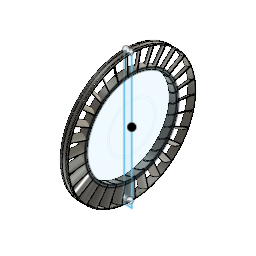
petrol_turbine_two_eng_model (Autodesk Fusion 360 design; units mm, degrees)
Autodesk Fusion 360 part; units mm, degrees
sketch "Sketch1" plane through (0, 0, 0) normal (1, 0, 0) x (0, 1, 0)
  circle A0 centre (0, 0) radius 58.75
  circle A1 centre (0, 0) radius 63.75
  dimension "d1" = 117.5
  dimension "d2" = 5
  constraint coincident A0.centre A1.centre
  measures "d1" diameter of A0
  measures "d2" distance of A0 A1
extrude "Extrude1" add sketch "Sketch1" along normal blind 20 makes body 1
sketch "Sketch2" plane through (0, 0, 0) normal (0, 1, 0) x (1, 0, 0)
  line L0 (0, -63.75) -> (0, 63.75)
  line L1 (20, -63.75) -> (20, 63.75)
  line L2 (0, 0) -> (0, -268.9117) construction
  line L3 (20, 0) -> (20, -259.4819) construction
  line L4 (0, -166.64) -> (20, -166.64)
  line L5 (0, -166.64) -> (0, -168.64)
  line L6 (20, -166.64) -> (20, -168.64)
  arc A0 (4, -168.64) -> (6, -168.64) centre (5, -168.64) ccw
  line L7 (0, -168.64) -> (4, -168.64)
  arc A1 (14, -168.64) -> (16, -168.64) centre (15, -168.64) ccw
  line L8 (6, -168.64) -> (14, -168.64)
  line L9 (16, -168.64) -> (20, -168.64)
  dimension "d5" = 166.64
  dimension "d6" = 166.64
  dimension "d8" = 2
  dimension "d9" = 2
  dimension "d10" = 5
  dimension "d11" = 5
  constraint coincident L2.start origin
  constraint parallel L0 L2
  constraint midpoint L1 L3.start
  constraint parallel L1 L3
  constraint coincident L2 L4.start
  constraint coincident L3 L4.end
  constraint coincident A0.centre L7
  constraint coincident A1.centre L7
  constraint coincident A0.end L7
  constraint collinear L7 L8
  constraint coincident A1.end L8
  constraint collinear L8 L9
  measures "d5" distance of L3.start L4.end
  measures "d6" distance of L2.start L4.start
  measures "d8" diameter of A0
  measures "d9" diameter of A1
  measures "d10" distance of L5.end A0.centre
  measures "d11" distance of L3 A1.centre
revolve "Revolve1" add sketch "Sketch2" angle 360 about axis through (1.75, 0, 0) along (1, 0, 0) separate body makes body 2
sketch "Sketch3" plane through (0, 0, 0) normal (0, 1, 0) x (1, 0, 0)
  line L0 (20, 168.64) -> (20, -168.64)
  line L1 (0, 168.64) -> (0, -168.64)
  line L2 (20, 168.64) -> (16, 168.64)
  line L3 (20, -168.64) -> (16, -168.64)
  arc A0 (14, -168.64) -> (16, -168.64) centre (15, -168.64) ccw
  arc A1 (16, 168.64) -> (14, 168.64) centre (15, 168.64) ccw
  line L4 (14, 168.64) -> (6, 168.64)
  line L5 (14, -168.64) -> (6, -168.64)
  arc A2 (4, -168.64) -> (6, -168.64) centre (5, -168.64) ccw
  arc A3 (6, 168.64) -> (4, 168.64) centre (5, 168.64) ccw
  line L6 (4, 168.64) -> (0, 168.64)
  line L7 (4, -168.64) -> (0, -168.64)
  line L8 (0, 168.64) -> (0, 183.603)
  line L9 (20, 168.64) -> (20, 183.603)
  line L10 (0, 183.603) -> (20, 183.603)
  constraint perpendicular L6 L8
  constraint perpendicular L2 L9
  constraint perpendicular L9 L10
sketch "Sketch4" plane through (0, 0, 0) normal (0, 0, 1) x (1, 0, 0)
  line L0 (0, 0) -> (74.0106, 0) construction
  line L1 (20, 168.64) -> (20, -168.64) construction
  line L2 (20, 0) -> (16, 0) construction
  arc A0 (19.8633, -9.4953) -> (2.0217, 0.9998) centre (1.5616, -20.1952) ccw
  arc A1 (18.1367, -10.5047) -> (1.9783, -0.9998) centre (1.5616, -20.1952) ccw
  line L3 (1.9783, -0.9998) -> (2.0217, 0.9998)
  line L4 (18.1367, -10.5047) -> (19.8633, -9.4953)
  point P0 (2, 0)
  point P1 (19, -10)
  dimension "d13" = 2
  dimension "d14" = 1
  dimension "d15" = 10
  constraint coincident L0.start origin
  constraint horizontal L0
  constraint coincident L0 P0
  measures "d13" distance of L0.start P0
  measures "d14" distance of P1 L1
  measures "d15" distance of P1 L2
extrude "Extrude2" add sketch "Sketch4" along normal blind 168 separate body makes body 3
fillet "Fillet1" radius 1 4 edges at (19.8633, -9.4953, 84) (18.1367, -10.5047, 84) (1.9783, -0.9998, 84) (2.0217, 0.9998, 84) on bodies 3
pattern_circular "C-Pattern1" count 30 over 360 about axis through (1.75, 0, 0) along (1, 0, 0) of bodies 3 makes body 4 at (18.7858, -30.9502, 107.9235) makes body 5 at (12.7085, -24.7526, 50.2791) makes body 6 at (17.0154, -70.4292, 87.2698) makes body 7 at (18.7858, -88.4751, 69.1198) makes body 8 at (14.9779, -98.8851, 52.726) makes body 9 at (18.2274, -108.7099, 27.8649) makes body 10 at (14.9779, -111.7816, 7.9474) makes body 11 at (18.7858, -110.5674, -19.4996) makes body 12 at (18.2274, -104.3268, -41.3549) makes body 13 at (18.2274, -93.4488, -62.1419) makes body 14 at (11.9072, -82.1008, -76.1992) makes body 15 at (14.9779, -62.7734, -92.8321) makes body 16 at (16.3643, -40.9695, -104.3585) makes body 17 at (11.9072, -21.6321, -109.9041) makes body 18 at (11.9072, 1.6909, -112) makes body 19 at (18.2274, 30.2232, -108.078) makes body 20 at (16.3643, 50.1395, -100.2757) makes body 21 at (18.2274, 71.5696, -86.4413) makes body 22 at (12.7085, 84.6791, -73.3357) makes body 23 at (16.3643, 99.5043, -51.6535) makes body 24 at (18.2274, 108.7099, -27.8649) makes body 25 at (14.9779, 111.7816, -7.9474) makes body 26 at (18.2274, 110.6451, 18.7604) makes body 27 at (14.9779, 105.3501, 38.2054) makes body 28 at (14.9779, 95.1046, 59.274) makes body 29 at (11.9072, 82.1008, 76.1992) makes body 30 at (14.9779, 62.7734, 92.8321) makes body 31 at (14.9779, 42.1008, 103.8548) makes body 32 at (16.3643, 18.3769, 110.596)
sketch "Sketch5" plane through (20, 0, 0) normal (1, 0, 0) x (0, 1, 0)
  circle A0 centre (0, 0) radius 58.75
  circle A1 centre (0, 0) radius 63.75
  circle A2 centre (0, 0) radius 58.75
  dimension "d25" = 117.5
  constraint coincident A0.centre A1.centre
  measures "d25" diameter of A2
extrude "Extrude3" cut sketch "Sketch5" along normal mid plane 80 contours A0 A2 bodies 3 4 5 6 7 8 9 10 11 12 13 14 15 16 17 18 19 20 21 22 23 24 25 26 27 28 29 30 31 32
combine "Combine1" operation add target body 17 tool bodies 20 5 12 13 23 2 10 25 6 29 32 21 15 18 4 27 9 1 22 7 31 24 26 8 11 19 14 3 28 30 16
sketch "Sketch6" plane through (20, 0, 0) normal (1, 0, 0) x (0, 1, 0)
  circle A0 centre (0, 0) radius 58.75
  circle A1 centre (0, 0) radius 63.75
  circle A2 centre (0, 0) radius 117.5
  circle A3 centre (0, 0) radius 122.5
  dimension "d28" = 235
  dimension "d29" = 5
  constraint coincident A0.centre A1.centre
  constraint concentric A2 A3
  measures "d28" diameter of A2
  measures "d29" distance of A2 A3
extrude "Extrude4" cut sketch "Sketch6" along normal mid plane 80 contours A0 | A1 | A2 bodies 17
extrude "Extrude5" add sketch "Sketch6" against normal blind 20 separate body contours A3 makes body 33
equation "d28 = ( 117.5 * 2 ) * 1 mm"
